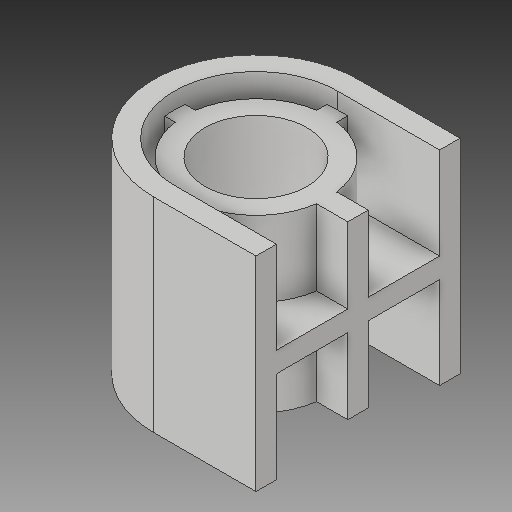
# Autodesk Inventor part: straight_beam_end_part_single
Saved by Autodesk Inventor 2019.3 (Build 233278000, 278)
## iProperties
Created: 2019-01-31
Part Number: straight_beam_end_part_single
Material: Generic
Document SubType Name: Modeling
Designer: Varga Daniel
Density: 1 g/cm^3
Appearance: Default
Author: Varga Daniel
Autodesk Inventor part; units mm, degrees
ref_plane "YZ Plane" through (0, 0, 0) normal (1, 0, 0) x (0, 1, 0)
ref_plane "XZ Plane" through (0, 0, 0) normal (0, 1, 0) x (-1, 0, 0)
ref_plane "XY Plane" through (0, 0, 0) normal (0, 0, 1) x (1, 0, 0)
derived "Base_part.ipt"
sketch "Sketch1" plane through (0, 0, 0) normal (0, 1, 0) x (-1, 0, 0)
  line L0 (5, 0) -> (25, 0)
  line L1 (30, 5) -> (30, 25)
  line L2 (25, 30) -> (5, 30)
  line L3 (0, 25) -> (0, 5)
  line L4 (5, 29) -> (25, 29)
  line L5 (29, 25) -> (29, 5)
  line L6 (25, 1) -> (5, 1)
  line L7 (1, 5) -> (1, 25)
  circle A0 centre (5, 5) radius 2.5
  circle A1 centre (5, 5) radius 3.5
  arc A2 (25, 0) -> (30, 5) centre (25, 5) ccw
  arc A3 (30, 25) -> (25, 30) centre (25, 25) ccw
  arc A4 (5, 30) -> (0, 25) centre (5, 25) ccw
  arc A5 (0, 5) -> (5, 0) centre (5, 5) ccw
  arc A6 (1, 5) -> (5, 1) centre (5, 5) ccw
  arc A7 (5, 29) -> (1, 25) centre (5, 25) ccw
  arc A8 (29, 25) -> (25, 29) centre (25, 25) ccw
  arc A9 (25, 1) -> (29, 5) centre (25, 5) ccw
  line L8 (49.1041, 15) -> (-27.081, 15) construction
  line L9 (31.1478, 10) -> (-2.4877, 10) construction
  line L10 (-2.8604, 5) -> (35.495, 5) construction
  line L11 (5, -2.5736) -> (5, 36.7522) construction
  line L12 (15, -1.4978) -> (15, 34.8784) construction
  line L13 (1.5359, 5.5) -> (1, 5.5)
  line L14 (1.5359, 4.5) -> (1.0314, 4.5)
  line L15 (28.9686, 4.5) -> (8.4641, 4.5)
  line L16 (29, 5.5) -> (8.4641, 5.5)
  line L17 (4.5, 1.5359) -> (4.5, 1.0314)
  line L18 (5.5, 1.5359) -> (5.5, 1)
  line L19 (29, 10.5) -> (1, 10.5)
  line L20 (29, 9.5) -> (1, 9.5)
  line L21 (4.5, 28.9686) -> (4.5, 10.5)
  line L22 (4.5, 9.5) -> (4.5, 8.4641)
  line L23 (5.5, 29) -> (5.5, 10.5)
  line L24 (5.5, 9.5) -> (5.5, 8.4641)
  point P0 (0, 0)
  point P1 (30, 30)
  point P2 (0, 30)
sketch "Sketch3" plane through (0, 0, 0) normal (0, 1, 0) x (-1, 0, 0)
  circle A0 centre (5, 5) radius 2.5 construction
  circle A1 centre (5, 5) radius 3.5 construction
  arc A2 (2.5, 5) -> (5, 7.5) centre (5, 5) ccw
  arc A3 (4.5, 1.5359) -> (5.5, 1.5359) centre (5, 5) ccw
  line L0 (0.3508, 5) -> (13.598, 5) construction
  line L1 (5, 13.9543) -> (5, -1.7484) construction
  line L2 (5, 10) -> (0, 10)
  line L3 (0, 10) -> (0, 9)
  line L4 (0, 9) -> (0, 9)
  line L5 (0, 1) -> (0, 0)
  line L6 (0, 0) -> (5, 0)
  line L7 (0, 0) -> (0, 1)
  line L8 (1.5359, 5.5) -> (0, 5.5)
  line L9 (0, 5.5) -> (0, 4.5)
  line L10 (0, 4.5) -> (1.5359, 4.5)
  line L11 (0, 9) -> (4.5, 9)
  line L12 (0, 9) -> (0, 10)
  line L13 (5, 9) -> (5, 9)
  line L14 (5, 1) -> (4.5, 1)
  arc A4 (5, 1) -> (5.5, 1.0314) centre (5, 5) ccw
  line L15 (4.5, 9) -> (4.5, 8.4641)
  line L16 (5.5, 8.9686) -> (5.5, 8.4641)
  line L17 (5.5, 1.0314) -> (5.5, 1.5359)
  line L18 (4.5, 1.5359) -> (4.5, 1)
  line L19 (8.4641, 5.5) -> (8.9686, 5.5)
  line L20 (8.4641, 4.5) -> (8.9686, 4.5)
  line L21 (0, 1) -> (0, 4.5)
  line L22 (0, 4.5) -> (0, 5.5)
  line L23 (0, 5.5) -> (0, 9)
  line L24 (4.5, 9) -> (5, 9)
  arc A5 (8.9686, 5.5) -> (5.5, 8.9686) centre (5, 5) ccw
  arc A6 (8.9686, 4.5) -> (8.9686, 5.5) centre (5, 5) ccw
  arc A7 (1.5359, 4.5) -> (4.5, 1.5359) centre (5, 5) ccw
  arc A8 (1.5359, 5.5) -> (1.5359, 4.5) centre (5, 5) ccw
  line L25 (4.5, 1) -> (0, 1)
  line L26 (0, 9) -> (4.5, 9)
  line L27 (4.5, 9) -> (5, 9)
  circle A9 centre (5, 5) radius 2.5 construction
  arc A10 (10, 5) -> (5, 10) centre (5, 5) ccw
  arc A11 (5, 0) -> (10, 5) centre (5, 5) ccw
  arc A12 (5.5, 8.9686) -> (5, 9) centre (5, 5) ccw
  arc A13 (8.4641, 5.5) -> (5.5, 8.4641) centre (5, 5) ccw
  arc A14 (5.5, 8.4641) -> (4.5, 8.4641) centre (5, 5) ccw
  arc A15 (5.5, 1.0314) -> (8.9686, 4.5) centre (5, 5) ccw
  arc A16 (8.4641, 4.5) -> (8.4641, 5.5) centre (5, 5) ccw
  arc A17 (4.5, 8.4641) -> (1.5359, 5.5) centre (5, 5) ccw
  arc A18 (5.5, 1.5359) -> (8.4641, 4.5) centre (5, 5) ccw
  arc A19 (5, 7.5) -> (2.5, 5) centre (5, 5) ccw
  point P0 (0, 0)
  dimension "d2" = 10
  dimension "d5" = 1
  dimension "d20" = 1
  dimension "d21" = 5
  dimension "d22" = 1
  dimension "d23" = 1
  dimension "d41" = 5
  dimension "d42" = 5
  dimension "d43" = 10
  constraints: 54 end point, 49 point on circle, 18 centre point, 14 perpendicular, 9 parallel, 9 point on line, 9 tangent, 5 collinear, 5 horizontal, 3 concentric, 2 coincident, 2 vertical, 12 other
  measures "d2" distance between parallel lines of L2 L6
  measures "d5" distance between parallel lines of L2 L4
  measures "d20" distance between parallel lines of L8 L10
  measures "d22" distance between parallel lines of L6 L14
  measures "d23" distance between parallel lines of L15 L16
  measures "d41" radius of A11
  measures "d42" radius of A10
  measures "d43" distance from line of A10.start L21
ref_plane "Work Plane2" through (0, 0, 5.5) normal (0, 1, 0) x (0, 0, 1)
extrude "Extrusion15" add sketch "Sketch3" along normal blind 5 contours L14 A4 A15 A6 A5 A12 L24 L11 L3 L2 A10 A11 L6 L5 L25
extrude "Extrusion16" add sketch "Sketch3" against normal blind 5 contours L14 A4 A15 A6 A5 A12 L24 L11 L3 L2 A10 A11 L6 L5 L25
extrude "Extrusion17" add sketch "Sketch3" along normal blind 4.2 contours A7 A8 A17 A14 A13 A16 A18 A3 | A3 L17 A4 L14 L18 | L10 L9 L8 A8 | A16 L19 A6 L20 | L15 L24 A12 L16 A14
extrude "Extrusion18" add sketch "Sketch3" against normal blind 4.2 contours A7 A8 A17 A14 A13 A16 A18 A3 | A3 L17 A4 L14 L18 | L10 L9 L8 A8 | A16 L19 A6 L20 | L15 L24 A12 L16 A14
extrude "Extrusion19" add sketch "Sketch3" along normal blind 0.5 contours L18 L25 L21 L10 A7 | A18 L20 A15 L17 | L8 L23 L11 L15 A17 | A13 L16 A5 L19
extrude "Extrusion20" add sketch "Sketch3" against normal blind 0.5 contours L18 L25 L21 L10 A7 | A18 L20 A15 L17 | L8 L23 L11 L15 A17 | A13 L16 A5 L19
equation "\"d5\" = Width_tolerance + Wall_thickness"
equation "\"d20\" = Inner_route_thickness"
equation "\"d22\" = Width_tolerance + Wall_thickness"
equation "\"d23\" = Inner_route_thickness"
equation "\"d44\" = 0.5 * Overall_height"
equation "\"d46\" = 0.5 * Overall_height"
equation "\"d48\" = 0.5 * Hole_height"
equation "\"d50\" = 0.5 * Hole_height"
equation "\"d52\" = 0.5 * Inner_thickness"
equation "\"d54\" = 0.5 * Inner_thickness"
equation "\"d4\" = Wall_thickness"
equation "\"d7\" = Inner_route_thickness"
equation "\"Width_tolerance\" = 0"
equation "\"Wall_thickness\" = 1"
equation "\"Inner_route_thickness\" = 1"
equation "\"Overall_height\" = 10"
equation "\"Hole_height\" = 8.4"
equation "\"Inner_thickness\" = 1"
body "Solid3"
